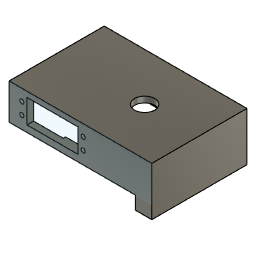
Chassis_Adv v6 (Autodesk Fusion 360 design; units mm, degrees)
Autodesk Fusion 360 part; units mm, degrees
note: some values were not read from the file. Set by a fixed rule: which sketch regions a step uses.
sketch "Sketch1" plane through (0, 0, 0) normal (1, 0, 0) x (0, 1, 0)
sketch "Sketch2" plane through (0, 0, 0) normal (0, 0, 1) x (1, 0, 0)
  line L0 (-60, -40) -> (60, -40)
  line L1 (60, -40) -> (60, 40)
  line L2 (60, 40) -> (-60, 40)
  line L3 (-60, 40) -> (-60, -40)
  line L4 (-60, -40) -> (60, 40) construction
  line L5 (60, -40) -> (-60, 40) construction
  dimension "d4" = 120
  dimension "d5" = 80
  constraint horizontal L0
  constraint perpendicular L0 L1
  constraint parallel L0 L2
  constraint parallel L1 L3
  constraint coincident L4 origin
  constraint coincident L5 origin
  measures "d4" distance of L1.end L2.end
  measures "d5" distance of L0.end L1.end
extrude "Extrude1" add sketch "Sketch2" along normal blind 30
sketch "Sketch9" plane through (0, 40, 0) normal (0, 1, 0) x (-1, 0, 0)
  line L0 (-60, 0) -> (60, 0)
  line L1 (60, 0) -> (60, 30)
  line L2 (60, 30) -> (-60, 30)
  line L3 (-60, 30) -> (-60, 0)
  line L4 (45, 5.5) -> (2, 5.5)
  line L5 (2, 5.5) -> (2, 25.5)
  line L6 (2, 25.5) -> (45, 25.5)
  line L7 (45, 25.5) -> (45, 5.5)
  line L8 (45, 5.5) -> (2, 25.5) construction
  line L9 (2, 5.5) -> (45, 25.5) construction
  line L10 (23.5, 15.5) -> (-4, 15.5) construction
  line L11 (23.5, 15.5) -> (51, 15.5) construction
  line L12 (-4, 25.5) -> (-4, 15.5) construction
  line L13 (2, 25.5) -> (-4, 25.5) construction
  line L14 (-4, 15.5) -> (-4, 20.5) construction
  line L15 (-4, 15.5) -> (-2.25, 15.5)
  line L16 (-4, 20.5) -> (-2.25, 20.5) construction
  circle A0 centre (-2.25, 20.5) radius 1.75
  circle A1 centre (-2.25, 10.5) radius 1.75
  line L17 (23.5, 5.5) -> (23.5, 25.5) construction
  circle A2 centre (49.25, 20.5) radius 1.75
  circle A3 centre (49.25, 10.5) radius 1.75
  point P0 (23.5, 15.5)
  dimension "d33" = 43
  dimension "d34" = 20
  dimension "d35" = 15
  dimension "d36" = 27.5
  dimension "d37" = 27.5
  dimension "d38" = 1.75
  dimension "d39" = 1.75
  dimension "d40" = 3.5
  constraint horizontal L4
  constraint perpendicular L4 L5
  constraint parallel L4 L6
  constraint parallel L5 L7
  constraint coincident L8 P0
  constraint coincident L9 P0
  constraint coincident P0 L10.start
  constraint perpendicular L5 L10
  constraint parallel L10 L11
  constraint perpendicular L10 L12
  constraint perpendicular L12 L13
  constraint midpoint L12 L14.end
  constraint perpendicular L14 L15
  constraint perpendicular L12 L16
  constraint coincident L16.end A0.centre
  constraint symmetric L10 A0 A1
  constraint midpoint L4 L17.start
  constraint midpoint L6 L17.end
  constraint symmetric A0 L17 A2
  constraint symmetric A1 L17 A3
  measures "d33" distance of L5.end L6.end
  measures "d34" distance of L4.end L5.end
  measures "d35" distance of L1 L4.start
  measures "d36" distance of P0 L10.end
  measures "d37" distance of P0 L11.end
  measures "d38" distance of L10.end L15.end
  measures "d39" distance of L14.end L16.end
  measures "d40" diameter of A0
extrude "Extrude5" cut sketch "Sketch9" against normal blind 133 contours L4 L5 L6 L7 | A0 | A1 | A2 | A3
sketch "Sketch10" plane through (0, 0, 0) normal (0, 0, 1) x (1, 0, 0)
  line L0 (0, 32.5) -> (-50, 32.5)
  line L1 (-50, 32.5) -> (-50, -32.5)
  line L2 (-50, -32.5) -> (0, -32.5)
  line L3 (0, -32.5) -> (0, 32.5)
  line L4 (60, 40) -> (-60, 40)
  dimension "d46" = 50
  dimension "d47" = 65
  dimension "d48" = 7.5
  constraint horizontal L0
  constraint vertical L1
  constraint horizontal L2
  constraint vertical L3
  measures "d46" distance of L0.start L0.end
  measures "d47" distance of L0.end L1.end
  measures "d48" distance of L0.end L4
extrude "Extrude6" cut sketch "Sketch10" along normal blind 25
extrude "Extrude7" cut 1 faces at (0, -10.8333, 8.3333) along direction (1, 0, 0) blind 30
move_body "Move1" bodies 1 to x (1, 0, 0) y (0, 1, 0) z (0, 0, 1) at (0, 0, 18.5)
sketch "Sketch11" plane through (0, 0, 18.5) normal (0, 0, -1) x (1, 0, 0)
  line L0 (30, -32.5) -> (-50, -32.5)
  line L1 (-50, -32.5) -> (-50, 32.5)
  line L2 (-50, 32.5) -> (30, 32.5)
  line L3 (30, 32.5) -> (30, -32.5)
  line L4 (-60, 40) -> (-60, -40)
  line L5 (-60, -40) -> (60, -40)
  line L6 (60, -40) -> (60, 40)
  line L7 (60, 40) -> (-60, 40)
  line L8 (30, 0) -> (40, 0) construction
  circle A0 centre (40, 0) radius 5
  line L9 (45, 0) -> (49.65, 0) construction
  line L10 (46.15, -30) -> (53.15, -30)
  line L11 (53.15, -30) -> (53.15, 30)
  line L12 (53.15, 30) -> (46.15, 30)
  line L13 (46.15, 30) -> (46.15, -30)
  line L14 (46.15, -30) -> (53.15, 30) construction
  line L15 (53.15, -30) -> (46.15, 30) construction
  point P0 (49.65, 0)
  dimension "d51" = 10
  dimension "d61" = 10
  dimension "d62" = 7
  dimension "d63" = 60
  constraint horizontal L8
  constraint coincident L8.end A0.centre
  constraint coincident A0 L9.start
  constraint horizontal L9
  constraint horizontal L10
  constraint perpendicular L10 L11
  constraint parallel L10 L12
  constraint parallel L11 L13
  constraint coincident L14 P0
  constraint coincident L15 P0
  constraint coincident P0 L9.end
  measures "d51" distance of L8.start L8.end
  measures "d61" diameter of A0
  measures "d62" distance of L11.end L12.end
  measures "d63" distance of L10.end L11.end
extrude "Extrude8" cut sketch "Sketch11" against normal blind 25 contours L10 L11 L12 L13
sketch "Sketch12" plane through (30, 0, 0) normal (-1, 0, 0) x (0, -1, 0)
  line L0 (-32.5, 18.5) -> (32.5, 18.5)
  line L1 (32.5, 18.5) -> (32.5, 43.5)
  line L2 (32.5, 43.5) -> (-32.5, 43.5)
  line L3 (-32.5, 43.5) -> (-32.5, 18.5)
  circle A0 centre (0, 30) radius 8.5
  dimension "d66" = 17
  measures "d66" diameter of A0
extrude "Extrude9" cut sketch "Sketch12" against normal blind 20 contours A0
sketch "Sketch13" plane through (0, 0, 18.5) normal (0, 0, -1) x (1, 0, 0)
  line L0 (53.15, -30) -> (46.15, -30)
  line L1 (46.15, -30) -> (46.15, 30)
  line L2 (46.15, 30) -> (53.15, 30)
  line L3 (53.15, 30) -> (53.15, -30)
  line L4 (30, -32.5) -> (-50, -32.5)
  line L5 (-50, -32.5) -> (-50, 32.5)
  line L6 (-50, 32.5) -> (30, 32.5)
  line L7 (30, 32.5) -> (30, -32.5)
  line L8 (-60, 40) -> (-60, -40)
  line L9 (-60, -40) -> (60, -40)
  line L10 (60, -40) -> (60, 40)
  line L11 (60, 40) -> (-60, 40)
  line L12 (53.15, 30) -> (60, 30)
  line L13 (60, -30) -> (53.15, -30)
  constraint coincident L2.end L3.start
  constraint coincident L10 L12.end
  constraint perpendicular L10 L12
  constraint coincident L10 L13.start
  constraint coincident L0.start L3.end
  constraint perpendicular L3 L13
extrude "Extrude10" add sketch "Sketch13" along normal blind 11 contours L3 L10 L12 L13
sketch "Sketch14" plane through (0, 0, 43.5) normal (0, 0, -1) x (1, 0, 0)
  line L0 (-2, 32.5) -> (-2, -32.5)
  line L1 (-2, -32.5) -> (30, -32.5)
  line L2 (30, -32.5) -> (30, 32.5)
  line L3 (30, 32.5) -> (-2, 32.5)
  circle A0 centre (14, 0) radius 8.5
  dimension "d71" = 17
  measures "d71" diameter of A0
extrude "Extrude11" cut sketch "Sketch14" against normal blind 5 contours A0
sketch "Sketch15" plane through (0, 0, 18.5) normal (0, 0, -1) x (1, 0, 0)
  line L0 (30, -32.5) -> (-50, -32.5)
  line L1 (-50, -32.5) -> (-50, 32.5)
  line L2 (-50, 32.5) -> (30, 32.5)
  line L3 (30, 32.5) -> (30, -32.5)
  line L4 (60, -30) -> (53.15, -30)
  line L5 (53.15, -30) -> (46.15, -30)
  line L6 (46.15, -30) -> (46.15, 30)
  line L7 (46.15, 30) -> (53.15, 30)
  line L8 (53.15, 30) -> (60, 30)
  line L9 (60, 30) -> (60, 40)
  line L10 (60, 40) -> (-60, 40)
  line L11 (-60, 40) -> (-60, -40)
  line L12 (-60, -40) -> (60, -40)
  line L13 (60, -40) -> (60, -30)
  line L14 (30, 0) -> (46.15, 0) construction
  circle A0 centre (38.075, 0) radius 6.75
  dimension "d74" = 13.5
  constraint midpoint L3 L14.start
  constraint midpoint L6 L14.end
  constraint midpoint L14 A0.centre
  measures "d74" diameter of A0
sketch "Sketch16" plane through (0, -40, 0) normal (0, -1, 0) x (1, 0, 0)
  circle A0 centre (2.25, 29) radius 1.75
  circle A1 centre (2.25, 39) radius 1.75
  circle A2 centre (-49.25, 39) radius 1.75
  line L0 (-2, 44) -> (-2, 24)
  line L1 (-2, 24) -> (-45, 24)
  line L2 (-45, 24) -> (-45, 44)
  line L3 (-45, 44) -> (-2, 44)
  circle A3 centre (-49.25, 29) radius 1.75
  line L4 (-60, 18.5) -> (60, 18.5)
  line L5 (60, 18.5) -> (60, 48.5)
  line L6 (60, 48.5) -> (-60, 48.5)
  line L7 (-60, 48.5) -> (-60, 18.5)
extrude "Extrude12" add sketch "Sketch15" along normal blind 18.5 contours A0
fillet "Fillet1" radius 5 1 faces at (40.0089, 2.266, 0)
sketch "Sketch17" plane through (0, 0, 18.5) normal (0, 0, -1) x (1, 0, 0)
  circle A0 centre (38.075, 0) radius 6.75
  line L0 (30, -32.5) -> (-50, -32.5)
  line L1 (-50, -32.5) -> (-50, 32.5)
  line L2 (-50, 32.5) -> (30, 32.5)
  line L3 (30, 32.5) -> (30, -32.5)
  line L4 (60, -30) -> (53.15, -30)
  line L5 (53.15, -30) -> (46.15, -30)
  line L6 (46.15, -30) -> (46.15, 30)
  line L7 (46.15, 30) -> (53.15, 30)
  line L8 (53.15, 30) -> (60, 30)
  line L9 (60, 30) -> (60, 40)
  line L10 (60, 40) -> (-60, 40)
  line L11 (-60, 40) -> (-60, -40)
  line L12 (-60, -40) -> (60, -40)
  line L13 (60, -40) -> (60, -30)
  line L14 (46.15, 30) -> (60, 30)
  line L15 (60, 30) -> (60, 40)
  line L16 (60, 40) -> (46.15, 40)
  line L17 (46.15, 40) -> (46.15, 30)
  line L18 (46.15, -30) -> (60, -30)
  line L19 (60, -30) -> (60, -40)
  line L20 (60, -40) -> (46.15, -40)
  line L21 (46.15, -40) -> (46.15, -30)
  constraint horizontal L14
  constraint vertical L15
  constraint horizontal L16
  constraint vertical L17
  constraint coincident L9.end L10.start
  constraint coincident L6.end L7.start
  constraint horizontal L18
  constraint vertical L19
  constraint horizontal L20
  constraint vertical L21
  constraint coincident L12.end L13.start
  constraint coincident L5.end L6.start
extrude "Extrude13" add sketch "Sketch17" along normal blind 11 contours L4 L5 L12 L13 L18 L19 L20 L21 | L7 L8 L9 L10 L14 L15 L16 L17
sketch "Sketch18" plane through (-60, 0, 0) normal (-1, 0, 0) x (0, -1, 0)
  line L0 (-40, 18.5) -> (40, 18.5)
  line L1 (40, 18.5) -> (40, 48.5)
  line L2 (40, 48.5) -> (-40, 48.5)
  line L3 (-40, 48.5) -> (-40, 18.5)
  line L4 (-35.5788, 18.5) -> (-35.5788, 43.0714)
  line L5 (-35.5788, 43.0714) -> (34.4212, 43.0714)
  line L6 (34.4212, 43.0714) -> (34.4212, 18.5)
  dimension "d82" = 70
  constraint coincident L0 L4.start
  constraint perpendicular L0 L4
  constraint perpendicular L4 L5
  constraint coincident L0 L6.end
  constraint perpendicular L0 L6
  measures "d82" distance of L4.end L5.end
extrude "Extrude14" cut sketch "Sketch18" against normal blind 40 contours L0 L4 L5 L6
